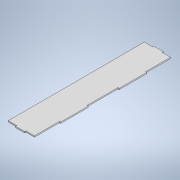
# Autodesk Inventor part: стенка боковая
Saved by Autodesk Inventor 2021 (Build 250183000, 183)
## iProperties
Created: 2023-02-14
Part Number: стенка боковая
Material: Типовые
Document SubType Name: Modeling
Designer: Tasya
Density: 1 g/cm^3
Appearance: По умолчанию
Author: Tasya
Autodesk Inventor part; units mm, degrees
ref_plane "YZ Plane" through (0, 0, 0) normal (1, 0, 0) x (0, 1, 0)
ref_plane "XZ Plane" through (0, 0, 0) normal (0, 1, 0) x (-1, 0, 0)
ref_plane "XY Plane" through (0, 0, 0) normal (0, 0, 1) x (1, 0, 0)
sketch "Эскиз1" plane through (0, 0, 0) normal (0, 1, 0) x (-1, 0, 0)
  line L0 (-42.5, 221) -> (42.5, 221)
  line L1 (42.5, 221) -> (42.5, -221)
  line L2 (42.5, -221) -> (-42.5, -221)
  line L3 (-42.5, -221) -> (-42.5, 221)
  line L4 (-42.5, 221) -> (42.5, -221) construction
  line L5 (42.5, 221) -> (-42.5, -221) construction
  line L6 (-42.5, 140) -> (-42.5, 50)
  line L7 (-42.5, 50) -> (-46.5, 50)
  line L8 (-46.5, 50) -> (-46.5, 140)
  line L9 (-46.5, 140) -> (-42.5, 140)
  line L10 (0, 0) -> (-15, 0) construction
  line L11 (-46.5, -50) -> (-46.5, -140)
  line L12 (-46.5, -140) -> (-42.5, -140)
  line L13 (-42.5, -50) -> (-46.5, -50)
  line L14 (-42.5, -140) -> (-42.5, -50)
  line L15 (-42.5, -24) -> (-42.5, 66)
  line L16 (15, 225) -> (15, 221)
  line L17 (15, 221) -> (-15, 221)
  line L18 (-15, 221) -> (-15, 225)
  line L19 (-15, 225) -> (15, 225)
  line L20 (15, 225) -> (-15, 221) construction
  line L21 (15, 221) -> (-15, 225) construction
  line L22 (0, 0) -> (0, 26.5579) construction
  line L23 (15, -225) -> (15, -221)
  line L24 (15, -221) -> (-15, -221)
  line L25 (-15, -221) -> (-15, -225)
  line L26 (-15, -225) -> (15, -225)
  point P0 (-10, -165.5)
  point P1 (-10, -255.5)
  point P2 (-10, -45)
  point P3 (-10, 45)
  point P4 (-42.5, -50)
  point P5 (-42.5, -140)
  point P6 (0, 223)
  point P7 (0, 223)
  point P8 (-15, -221)
  point P9 (15, -221)
  dimension "d0" = 442
  dimension "d1" = 85
  dimension "d2" = 4
  dimension "d3" = 90
  dimension "d4" = 50
  dimension "d9" = 30
  dimension "d11" = 4
  constraints: 54 end point, 8 symmetric about line, 6 midpoint, 6 parallel, 3 perpendicular, 3 point on line, 2 collinear, 2 horizontal, 2 vertical, 1 coincident
  measures "d0" distance of L2.end L0.start
  measures "d1" distance between parallel lines of L3 L1
  measures "d2" distance of L6.end L7.end
  measures "d3" distance of L7.end L8.end
  measures "d4" distance between parallel lines of L10 L7
  measures "d9" distance of L18.end L16.start
  measures "d11" distance of L17.end L18.end
extrude "Выдавливание1" add sketch "Эскиз1" along normal blind 4
